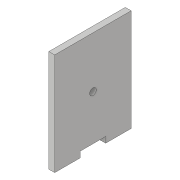
# Autodesk Inventor part: wheelsupport
Saved by Autodesk Inventor 2017 (Build 210142000, 142)
## iProperties
Created: 2019-06-10
Part Number: wheelsupport
Material: Generic
Document SubType Name: Modeling
Designer: markg
Density: 1 g/cm^3
Appearance: Default
Author: markg
Autodesk Inventor part; units mm, degrees
ref_plane "YZ Plane" through (0, 0, 0) normal (1, 0, 0) x (0, 1, 0)
ref_plane "XZ Plane" through (0, 0, 0) normal (0, 1, 0) x (-1, 0, 0)
ref_plane "XY Plane" through (0, 0, 0) normal (0, 0, 1) x (1, 0, 0)
sketch "Sketch1" plane through (0, 0, 0) normal (1, 0, 0) x (0, 1, 0)
  line L0 (0, 0) -> (50.8, 0)
  line L1 (50.8, 0) -> (50.8, -38.1)
  line L2 (50.8, -38.1) -> (0, -38.1)
  circle A0 centre (25.4, -19.05) radius 1.651
  line L3 (0, -12.7) -> (2.921, -12.7)
  line L4 (2.921, -12.7) -> (2.921, -25.4)
  line L5 (2.921, -25.4) -> (0, -25.4)
  line L6 (0, -38.1) -> (0, -25.4)
  line L7 (0, -12.7) -> (0, 0)
  dimension "d0" = 50.8
  dimension "d1" = 38.1
  dimension "d2" = 3.302
  dimension "d9" = 12.7
  dimension "d10" = 12.7
  dimension "d11" = 2.921
  constraints: 16 end point, 4 parallel, 2 horizontal, 2 perpendicular, 1 centre point
  measures "d0" distance of L1.end L2.end
  measures "d1" distance of L0.end L1.end
  measures "d2" diameter of A0
  measures "d9" distance of L3.start L0.start
  measures "d10" distance of L2.end L5.end
  measures "d11" distance of L4.end L5.end
extrude "Extrusion1" add sketch "Sketch1" along normal blind 2.921
body "Solid1"
